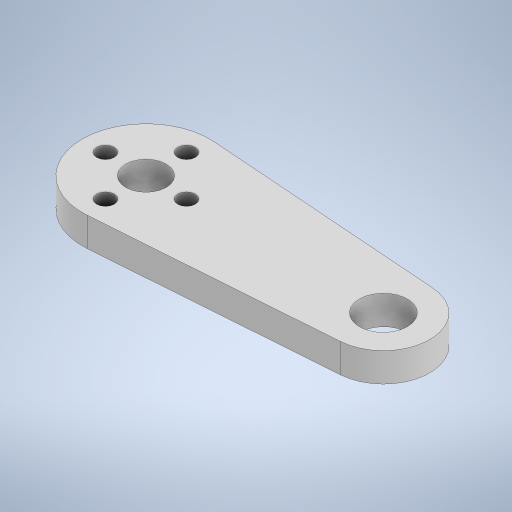
# Autodesk Inventor part: leg4
Saved by Autodesk Inventor 2024 (Build 280153000, 153)
## iProperties
Created: 2023-08-18
Part Number: leg4
Material: 常规
Document SubType Name: Modeling
Designer: wya
Density: 1 g/cm^3
Appearance: 默认
Author: wya
Autodesk Inventor part; units mm, degrees
ref_plane "YZ Plane" through (0, 0, 0) normal (1, 0, 0) x (0, 1, 0)
ref_plane "XZ Plane" through (0, 0, 0) normal (0, 1, 0) x (-1, 0, 0)
ref_plane "XY Plane" through (0, 0, 0) normal (0, 0, 1) x (1, 0, 0)
sketch "草图1" plane through (0, 0, 0) normal (0, 1, 0) x (-1, 0, 0)
  circle A0 centre (0, 0) radius 11
  circle A1 centre (0, 0) radius 3.5
  circle A2 centre (0, 0) radius 7
  circle A3 centre (7, 0) radius 1.525
  circle A4 centre (0, 7) radius 1.525
  circle A5 centre (-7, 0) radius 1.525
  circle A6 centre (0, -7) radius 1.525
  line L0 (0, 0) -> (2.6058, 0)
  line L1 (0, 0) -> (0, -1.55)
  line L2 (-0.8049, 10.9705) -> (-41.5854, 7.9786)
  line L3 (-41.5854, 7.9786) -> (-41.5854, -7.9786)
  line L4 (-41.5854, -7.9786) -> (-0.8049, -10.9705)
  circle A7 centre (-41, 0) radius 8
  circle A8 centre (-41, 0) radius 4.15
  point P0 (-41.5854, -7.9786)
  dimension "d7" = 16
  dimension "d0" = 22
  dimension "d1" = 7
  dimension "d2" = 14
  dimension "d3" = 3.05
  dimension "d4" = 3.05
  dimension "d5" = 3.05
  dimension "d6" = 3.05
  dimension "d8" = 41
  dimension "d9" = 8.3
  constraints: 10 end point, 8 centre point, 6 point on circle, 4 coincident, 4 point on line, 2 tangent, 2 vertical, 1 equal length, 1 horizontal, 5 other
  measures "d0" diameter of A0
  measures "d1" diameter of A1
  measures "d2" diameter of A2
  measures "d3" diameter of A3
  measures "d4" diameter of A4
  measures "d5" diameter of A5
  measures "d6" diameter of A6
  measures "d8" distance of point (-41, 0) A0.centre
  measures "d9" diameter of A8
extrude "拉伸1" add sketch "草图1" along normal blind 5 contours A0 | A0 L4 A7 L2 | A7 L3 A8 | L3 A8 A7 | A3 A2 A6 A5 A4
